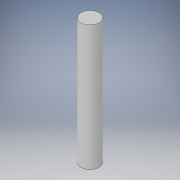
# Autodesk Inventor part: rope hole straight
Saved by Autodesk Inventor 2019 (Build 230136000, 136)
## iProperties
Created: 2018-09-12
Part Number: rope hole straight
Material: Generic
Document SubType Name: Modeling
Designer: HIVE
Density: 1 g/cm^3
Appearance: Default
Author: HIVE
## iProperties of the stored document rope hole straight_3DPrint.ipt
Created: 2018-09-12
Part Number: rope hole straight_3DPrint
Material: Generic
Document SubType Name: Modeling
Designer: HIVE
Density: 1 g/cm^3
Appearance: Default
Author: HIVE
Autodesk Inventor part; units mm, degrees
ref_plane "YZ Plane" through (0, 0, 0) normal (1, 0, 0) x (0, 1, 0)
ref_plane "XZ Plane" through (0, 0, 0) normal (0, 1, 0) x (-1, 0, 0)
ref_plane "XY Plane" through (0, 0, 0) normal (0, 0, 1) x (1, 0, 0)
sketch "Sketch1" plane through (0, 0, 0) normal (0, 1, 0) x (-1, 0, 0)
  circle A0 centre (0, 0) radius 2.5
  dimension "d0" = 5
  constraints: 1 centre point, 1 coincident
  measures "d0" diameter of A0
extrude "Extrusion1" add sketch "Sketch1" along normal blind 35
body "Solid1"
